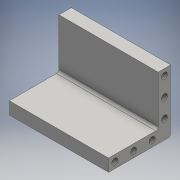
# Autodesk Inventor part: Profile_Middle_02
Saved by Autodesk Inventor 2016 (Build 200138000, 138)
## iProperties
Created: 2016-02-09
Part Number: Profile_Middle_02
Material: Generic
Document SubType Name: Modeling
Designer: nils
Density: 1 g/cm^3
Appearance: Default
Author: nils
Autodesk Inventor part; units mm, degrees
ref_plane "YZ Plane" through (0, 0, 0) normal (1, 0, 0) x (0, 1, 0)
ref_plane "XZ Plane" through (0, 0, 0) normal (0, 1, 0) x (-1, 0, 0)
sketch "Sketch2" plane through (0, 0, 0) normal (1, 0, 0) x (0, 1, 0)
  line L0 (0, 0) -> (50, 0)
  line L1 (50, 0) -> (50, -50)
  line L2 (50, -50) -> (0, -50)
  line L3 (0, -50) -> (0, 0)
  line L4 (0, 0) -> (40, 0)
  line L5 (40, 0) -> (40, -40)
  line L6 (40, -40) -> (0, -40)
  line L7 (0, -40) -> (0, 0)
  dimension "d5" = 50
  dimension "d6" = 50
  dimension "d7" = 10
  dimension "d8" = 10
  constraints: 16 end point, 4 parallel, 2 horizontal, 2 perpendicular
  measures "d5" distance of L1.end L2.end
  measures "d6" distance of L0.end L1.end
  measures "d7" distance between parallel lines of L5 L1
  measures "d8" distance between parallel lines of L2 L6
extrude "Extrusion1" add sketch "Sketch2" along normal blind 80 contours L0 L1 L2 L3 L6 L5
fillet "Fillet1" radius 2 2 edges at (40, 40, -40) (40, 50, -50)
sketch "Sketch6" plane through (0, 0, 0) normal (-1, 0, 0) x (0, 0, 1)
  line L0 (-40, 0) -> (-50, 0) projected
  line L1 (-45, 0) -> (-45, 50)
  line L2 (-48, 50) -> (0, 50) projected
  line L3 (0, 50) -> (0, 40) projected
  line L4 (0, 45) -> (-50, 45)
  point P0 (0, 0)
  point P1 (-50, 50)
  point P2 (-5, 45)
  point P3 (-20, 45)
  point P4 (-35, 45)
  point P5 (-45, 35)
  point P6 (-45, 5)
  point P7 (-45, 20)
  dimension "d23" = 5
  dimension "d25" = 20
  dimension "d26" = 35
  dimension "d27" = 5
  dimension "d28" = 20
  dimension "d29" = 35
  constraints: 7 point on line, 4 end point, 2 midpoint, 1 parallel, 1 vertical
  measures "d23" distance from line of L0 point (-45, 5)
  measures "d25" distance from line of L0 point (-45, 20)
  measures "d26" distance from line of L0 point (-45, 35)
  measures "d27" distance from line of L3 point (-5, 45)
  measures "d28" distance from line of L3 point (-20, 45)
  measures "d29" distance from line of L3 point (-35, 45)
hole "Hole1" at (0, 45, -5) at (0, 45, -20) at (0, 45, -35) at (0, 35, -45) at (0, 5, -45) at (0, 20, -45) direction (1, 0, 0) diameter 4.917 depth 17.1 tip angle 118 thread size "M6x1" class "6H" standard "ISO Metric profile"
ref_plane "Work Plane1" through (40, 0, 0) normal (-1, 0, 0) x (0, 0, 1)
mirror "Mirror1" about plane through (40, 0, 0) normal (-1, 0, 0) of "Hole1"
ref_plane "Work Plane2" through (40, 0, 0) normal (-1, 0, 0) x (0, 0, 1)
body "Solid1"
